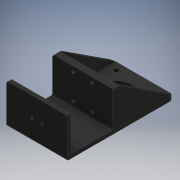
# Autodesk Inventor part: Extruder_Mount
Saved by Autodesk Inventor 2017.3 (Build 213256000, 256)
## iProperties
Created: 2018-09-09
Part Number: Extruder_Mount
Material: ABS Plastic
Document SubType Name: Modeling
Designer: Ax
Density: 1.06 g/cm^3
Appearance: 0,0,0
Author: Ax
## iProperties of the stored document Extruder_Mount_3DPrint.ipt
Created: 2018-09-09
Part Number: Extruder_Mount_3DPrint
Material: Generic
Document SubType Name: Modeling
Designer: Ax
Density: 1 g/cm^3
Appearance: Default
Author: Ax
Autodesk Inventor part; units mm, degrees
ref_plane "YZ Plane" through (0, 0, 0) normal (1, 0, 0) x (0, 1, 0)
ref_plane "XZ Plane" through (0, 0, 0) normal (0, 1, 0) x (-1, 0, 0)
ref_plane "XY Plane" through (0, 0, 0) normal (0, 0, 1) x (1, 0, 0)
sketch "Sketch1" plane through (0, 0, 0) normal (1, 0, 0) x (0, 1, 0)
  line L0 (0, 0) -> (84.4, 0)
  line L1 (84.4, 0) -> (84.4, 3)
  line L2 (84.4, 3) -> (41.4, 3)
  line L3 (41.4, 3) -> (41.4, 31)
  line L4 (41.4, 31) -> (36.4, 31)
  line L5 (36.4, 31) -> (36.4, 3)
  line L6 (36.4, 3) -> (3, 3)
  line L7 (3, 3) -> (3, 31)
  line L8 (3, 31) -> (0, 31)
  line L9 (0, 31) -> (0, 0)
  line L10 (0, 0) -> (84.4, 0)
  dimension "d0" = 3
  dimension "d1" = 5
  dimension "d2" = 33.4
  dimension "d3" = 43
  dimension "d4" = 28
  constraints: 22 end point, 9 perpendicular, 2 equal length, 2 point on line, 1 horizontal
  measures "d0" distance of L0.end L1.end
  measures "d1" distance of L3.end L4.end
  measures "d2" distance of L5.end L6.end
  measures "d3" distance of L1.end L2.end
  measures "d4" distance of L2.end L3.end
extrude "Extrusion1" add sketch "Sketch1" along normal mid plane 48
sketch "Sketch2" plane through (24, 0, 0) normal (1, 0, 0) x (0, 0, -1)
  line L0 (0, 0) -> (0, 84.4) projected
  line L1 (-3, 41.4) -> (-31, 41.4) projected
  line L2 (-3, 41.4) -> (-31, 41.4)
  line L3 (-3, 84.4) -> (-3, 41.4) projected
  line L4 (-3, 41.4) -> (-3, 84.4)
  line L5 (-3, 84.4) -> (-31, 41.4)
  constraints: 6 end point, 2 collinear
extrude "Extrusion2" add sketch "Sketch2" against normal blind 2
sketch "Sketch3" plane through (-24, 0, 0) normal (-1, 0, 0) x (0, 0, 1)
  line L0 (31, 41.4) -> (3, 41.4) projected
  line L1 (31, 41.4) -> (3, 41.4)
  line L2 (0, 0) -> (0, 84.4) projected
  line L3 (3, 41.4) -> (3, 84.4) projected
  line L4 (3, 41.4) -> (3, 84.4)
  line L5 (3, 84.4) -> (31, 41.4)
  constraints: 6 end point, 2 collinear
extrude "Extrusion3" add sketch "Sketch3" against normal blind 2
sketch "Sketch10" plane through (22, 41.4, 3) normal (0, 0, 1) x (1, 0, 0)
  line L0 (0, 0) -> (0, 43) construction
  line L1 (-46, 43) -> (2, 43) construction
  line L2 (-44, 0) -> (0, 0) construction
  line L3 (-6.5, 6) -> (-37.5, 6) construction
  line L4 (-37.5, 6) -> (-37.5, 37) construction
  line L5 (-37.5, 37) -> (-6.5, 37) construction
  line L6 (-6.5, 37) -> (-6.5, 6) construction
  circle A0 centre (-22, 21.5) radius 12
  circle A1 centre (-6.5, 6) radius 1.7
  circle A2 centre (-37.5, 6) radius 1.7
  circle A3 centre (-37.5, 37) radius 1.7
  circle A4 centre (-6.5, 37) radius 1.7
  line L7 (0, 21.5) -> (-44, 21.5) construction
  line L8 (0, 0) -> (0, 43) construction
  line L9 (-44, 43) -> (-44, 0) construction
  line L10 (-22, 43) -> (-22, 0) construction
  point P0 (-22, -41.4)
  point P1 (-22, 21.5)
  dimension "d26" = 31
  dimension "d27" = 24
  dimension "d28" = 3.4
  constraints: 12 end point, 8 midpoint, 5 centre point, 4 coincident, 3 equal radius, 3 perpendicular, 2 horizontal, 2 parallel, 2 symmetric about line
  measures "d26" distance of L4.end L5.end
  measures "d27" diameter of A0
  measures "d28" diameter of A2
extrude "Extrusion4" cut sketch "Sketch10" against normal through all
sketch "Sketch11" plane through (22, 41.4, 31) normal (0, 1, 0) x (1, 0, 0)
  line L0 (0, 0) -> (-44, 28) construction
  line L1 (-44, 0) -> (0, 28) construction
  line L2 (-14.5, 24) -> (-29.5, 24) construction
  line L3 (-29.5, 24) -> (-29.5, 4) construction
  line L4 (-29.5, 4) -> (-14.5, 4) construction
  line L5 (-14.5, 4) -> (-14.5, 24) construction
  line L6 (-14.5, 24) -> (-29.5, 4) construction
  line L7 (-29.5, 24) -> (-14.5, 4) construction
  circle A0 centre (-14.5, 4) radius 1.7
  circle A1 centre (-29.5, 4) radius 1.7
  circle A2 centre (-29.5, 24) radius 1.7
  circle A3 centre (-14.5, 24) radius 1.7
  point P0 (-44, 0)
  point P1 (-22, 14)
  dimension "d32" = 20
  dimension "d33" = 15
  dimension "d34" = 3.4
  constraints: 16 end point, 8 coincident, 4 centre point, 3 equal radius, 3 midpoint, 2 parallel, 1 horizontal, 1 perpendicular
  measures "d32" distance of L2.end L3.end
  measures "d33" distance of L3.end L4.end
  measures "d34" diameter of A1
hole "Hole1" at (7.5, 41.4, 27) at (-7.5, 41.4, 27) at (-7.5, 41.4, 7) at (7.5, 41.4, 7) direction (0, -1, 0) diameter 2.459 depth 8.8 tip angle 118 countersink diameter 4 countersink angle 90 thread size "M3x0.5" class "6H" standard "ISO Metric profile"
sketch "Sketch12" plane through (-24, 0, 0) normal (0, -1, 0) x (1, 0, 0)
  line L0 (24, 31) -> (24, 0) construction
  line L1 (0, 0) -> (48, 0) construction
  line L2 (0, 31) -> (48, 31) construction
  line L3 (0, 15.5) -> (48, 15.5) construction
  line L4 (0, 0) -> (0, 31) construction
  line L5 (48, 31) -> (48, 0) construction
  circle A0 centre (20, 15.5) radius 1.5
  circle A1 centre (28, 15.5) radius 1.5
  dimension "d42" = 3
  dimension "d43" = 8
  constraints: 4 end point, 3 midpoint, 2 centre point, 2 point on line, 2 symmetric about line, 1 equal radius, 1 horizontal, 1 perpendicular
  measures "d42" diameter of A1
  measures "d43" distance of A1.centre A0.centre
hole "Hole2" at (-4, 0, 15.5) at (4, 0, 15.5) direction (0, 1, 0) diameter 2.459 depth 8.8 thread size "M3x0.5" class "6H" standard "ISO Metric profile"
fillet "Fillet1" radius 3 2 edges at (-24, 84.4, 1.5) (24, 84.4, 1.5)
fillet "Fillet2" radius 1 1 edges at (0, 0, 0)
fillet "Fillet3" radius 1 2 edges at (0, 36.4, 3) (0, 3, 3)
fillet "Fillet4" radius 2 4 edges at (24, 38.9, 31) (-24, 38.9, 31) (24, 1.5, 31) (-24, 1.5, 31)
body "Solid33"
